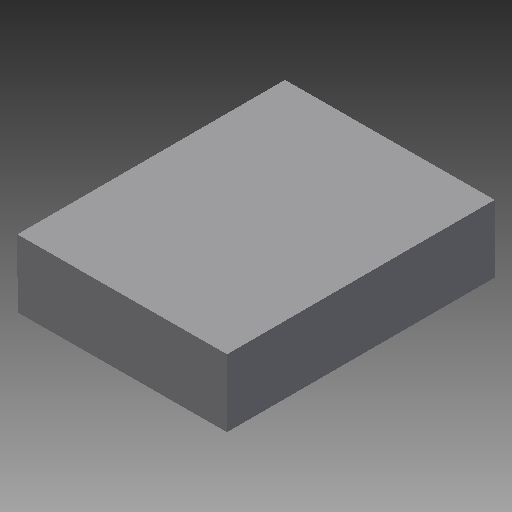
# Autodesk Inventor part: nzm1_3p_p3
Saved by Autodesk Inventor 2019.3 (Build 233278000, 278)
## iProperties
Category: PARTsolutions
Company: MOELLER
Created: 2018-10-25
Part Number: nzm1_3p_p3
Material: Generic
Catalog Web Link: www.cadenas.de
Description: Leistungsschalter 3p_p3-Leistungsschalter 3p
Vendor: MOELLER
Document SubType Name: Modeling
Designer: psadmin
Manufacturer: MOELLER
Mass: 0.626083 g
Surface Area: 5.32385 cm^2
Volume: 0.626083 cm^3
Density: 1 g/cm^3
Appearance: PSOLRGB-192-192-192
PSOL_IDENT_0: {$CADENAS_DATA\23d-libs\moeller\circuit_breaker\parts\nzm1_3p_p3.prj},178 {VTYP=3D},{NB=nzm1_3p_p3},
PSOL_IDENT_1: {LINA=nzm1_3p_p3},{NN=Leistungsschalter 3p_p3},{DATE=05.10.2018 14:14:12},{GEOMDATE=14.05.2018 10:43
PSOL_IDENT_2: :05},{VERSION=},{LINEID=310},{WBVAR=},{WBNUMERIC=}  {NB=nzm1_3p_p3},{LINA=nzm1_3p_p3},{KT=DUMMY},{BM
PSOL_IDENT_3: ENB=nzm1_3p_p3},{EPLAN=}
NN: Leistungsschalter 3p_p3
NT: Leistungsschalter 3p
NB: nzm1_3p_p3
NBSYN: $BMENB.
LINA: nzm1_3p_p3
BMENB: nzm1_3p_p3
SUPPLIER: MOELLER
ARTICLENO: nzm1_3p_p3
BOMINFO: nzm1_3p_p3
CREATOR: CADENAS GmbH
Title: nzm1_3p_p3
Author: Cadenas PARTsolutions
Comments: Leistungsschalter 3p
Autodesk Inventor part; units mm, degrees
sketch "Sketch_1" plane through (0, 0, 0) normal (0, 0, 1) x (1, 0, 0)
  line L0 (-11.519, 1.7998) -> (-11.5028, -1.9002)
  line L1 (-11.5028, -1.9002) -> (0, -1.85)
  line L2 (0, -1.85) -> (0, 1.85)
  line L3 (0, 1.85) -> (-11.519, 1.7998)
  constraints: 8 end point
extrude "Extrusion1" add sketch "Sketch_1" along normal mid plane 14.7
ref_plane "P3_XY" through (0, 0, 0) normal (1, 0, 0) x (0, 0, -1)
ref_plane "P3_YZ" through (0, 0, 0) normal (0, 0, -1) x (0, 1, 0)
ref_plane "P3_ZX" through (0, 0, 0) normal (0, 1, 0) x (1, 0, 0)
body "Solid1"
